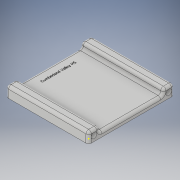
# Autodesk Inventor part: MousetrapHolder
Saved by Autodesk Inventor 2018 (Build 220112000, 112)
## iProperties
Created: 2018-09-22
Part Number: MousetrapHolder
Material: Generic
Document SubType Name: Modeling
Designer: Aditya Kendre
Density: 1 g/cm^3
Appearance: Default
Author: Aditya Kendre
Autodesk Inventor part; units mm, degrees
ref_plane "YZ Plane" through (0, 0, 0) normal (1, 0, 0) x (0, 1, 0)
ref_plane "XZ Plane" through (0, 0, 0) normal (0, 1, 0) x (-1, 0, 0)
ref_plane "XY Plane" through (0, 0, 0) normal (0, 0, 1) x (1, 0, 0)
sketch "Sketch1" plane through (0, 0, 0) normal (0, 1, 0) x (-1, 0, 0)
  line L0 (0, 0) -> (98.425, 0)
  line L1 (98.425, 0) -> (98.425, -101.6)
  line L2 (98.425, -101.6) -> (0, -101.6)
  line L3 (0, -101.6) -> (0, 0)
  dimension "d0" = 98.425
  dimension "d1" = 101.6
  constraints: 8 end point, 2 parallel, 1 horizontal, 1 perpendicular
  measures "d0" distance of L1.end L2.end
  measures "d1" distance of L0.end L1.end
extrude "Extrusion1" add sketch "Sketch1" along normal blind 6.35
sketch "Sketch2" plane through (0, 6.35, 0) normal (0, 1, 0) x (1, 0, 0)
  line L0 (-98.425, 0) -> (0, 0) projected
  line L1 (-98.425, 101.6) -> (-98.425, 0) projected
  line L2 (0, 0) -> (-98.425, 0)
  line L3 (-98.425, 0) -> (-98.425, 12.7)
  line L4 (-98.425, 12.7) -> (0, 12.7)
  line L5 (0, 12.7) -> (0, 0)
  line L6 (0, 0) -> (0, 101.6) projected
  line L7 (0, 101.6) -> (-98.425, 101.6)
  line L8 (-98.425, 101.6) -> (-98.425, 88.9)
  line L9 (-98.425, 88.9) -> (0, 88.9)
  line L10 (0, 88.9) -> (0, 101.6)
  dimension "d4" = 12.7
  dimension "d5" = 12.7
  constraints: 16 end point, 4 parallel, 2 horizontal, 2 perpendicular, 2 point on line
  measures "d4" distance of L2.end L3.end
  measures "d5" distance of L8.end L7.end
extrude "Extrusion2" add sketch "Sketch2" along normal blind 6.35 contours L1 L4 L5 L0 | L1 L7 L6 L9
sketch "Sketch3" plane through (0, 0, 0) normal (1, 0, 0) x (0, 0, -1)
  point P0 (0, 0)
  point P1 (6.35, 6.35)
  point P2 (95.25, 6.35)
hole "Hole1" at (0, 6.35, -6.35) at (0, 6.35, -95.25) direction (-1, 0, 0) diameter 6.604 end through all
fillet "Fillet1" radius 3.175 1 edges at (-49.2125, 6.35, -12.7)
fillet "Fillet2" radius 3.175 1 edges at (-49.2125, 6.35, -88.9)
fillet "Fillet3" radius 3.175 5 edges at (0, 6.35, -50.8) (0, 7.2799, -87.9701) (0, 11.1125, -88.9) (0, 7.2799, -13.6299) (0, 11.1125, -12.7)
fillet "Fillet4" radius 3.175 5 edges at (-98.425, 6.35, -50.8) (-98.425, 7.2799, -13.6299) (-98.425, 11.1125, -12.7) (-98.425, 7.2799, -87.9701) (-98.425, 11.1125, -88.9)
fillet "Fillet5" radius 3.175 1 edges at (-49.2125, 12.7, 0)
fillet "Fillet6" radius 3.175 9 edges at (-49.1878, 12.7, -12.7) (-97.4951, 12.7, -11.7701) (-98.425, 12.7, -6.35) (-98.425, 11.7701, -0.9299) (-98.425, 4.7625, 0) (-0.9299, 12.7, -11.7701) (0, 12.7, -6.3747) (0, 11.7701, -0.9299) (0, 4.7625, 0)
fillet "Fillet7" radius 3.175 5 edges at (-49.1878, 12.7, -88.9) (-0.9299, 12.7, -89.8299) (0, 12.7, -96.8128) (-97.4951, 12.7, -89.8299) (-98.425, 12.7, -96.8375)
fillet "Fillet8" radius 3.175 5 edges at (-49.2125, 12.7, -101.6) (-97.4951, 11.7701, -101.6) (-98.425, 4.7625, -101.6) (-0.9299, 11.7701, -101.6) (0, 4.7625, -101.6)
sketch "Sketch4" plane through (0, 6.35, 0) normal (0, 1, 0) x (1, 0, 0)
  line L0 (-88.3129, 30.0873) -> (-88.3129, 71.0032) construction
  line L1 (-88.3129, 71.0032) -> (-84.2868, 71.0032) construction
  line L2 (-84.2868, 71.0032) -> (-84.2868, 30.0873) construction
  line L3 (-84.2868, 30.0873) -> (-88.3129, 30.0873) construction
  point P0 (0, 0)
  constraints: 2 other
body "Solid1"
